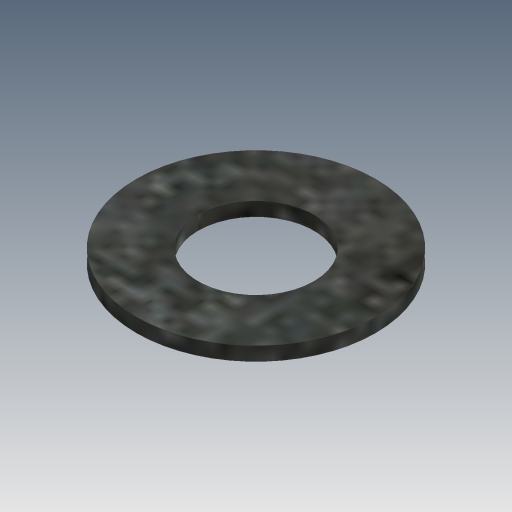
# Autodesk Inventor part: Metal Washer (RAM-201U-B)
Saved by Autodesk Inventor 2023.1 (Build 271208000, 208)
## iProperties
Created: 2023-01-24
Part Number: Metal Washer (RAM-201U-B)
Material: Acciaio
Document SubType Name: Modeling
Designer: Cominelli Nicolas
Mass: 1.87425 g
Surface Area: 5.31557 cm^2
Volume: 0.238758 cm^3
Density: 7.85 g/cm^3
Appearance: Lamiera
Author: Cominelli Nicolas
Costo: 0
Trattamento: -
Autodesk Inventor part; units mm, degrees
ref_plane "YZ Plane" through (0, 0, 0) normal (1, 0, 0) x (0, 1, 0)
ref_plane "XZ Plane" through (0, 0, 0) normal (0, 1, 0) x (-1, 0, 0)
ref_plane "XY Plane" through (0, 0, 0) normal (0, 0, 1) x (1, 0, 0)
sketch "Schizzo4" plane through (0, 0, 0) normal (0, 0, 1) x (1, 0, 0)
  line L0 (0, 0) -> (0, 1.1)
  line L1 (4.6, 0) -> (4.6, 1.1)
  line L2 (4.6, 1.1) -> (9.5, 1.1)
  line L3 (9.5, 1.1) -> (9.5, 0)
  line L4 (9.5, 0) -> (4.6, 0)
  dimension "d0" = 1.1
  dimension "d1" = 9.2
  dimension "d2" = 19
  constraints: 10 end point, 2 horizontal alignment, 2 perpendicular, 2 vertical, 1 horizontal
  measures "d0" distance between parallel lines of L4 L2
  measures "d1" diameter of L1 L0
  measures "d2" diameter of L3 L0
revolve "Rivoluzione1" add sketch "Schizzo4" angle 360 about axis through (0, 0, 0) along (0, 1, 0)
